rod_label_clip (Autodesk Fusion 360 design; units mm, degrees)
part number: 2026-09-05-07-00-16-324
Autodesk Fusion 360 part; units mm, degrees
sketch "Ring" plane through (0, 0, 0) normal (0, 1, 0) x (1, 0, 0)
  circle A0 centre (0, 0) radius 17.05
  circle A1 centre (0, 0) radius 19.45
  dimension "d32" = 34.1
  dimension "d33" = 38.9
  constraint coincident A0.centre A1.centre
  constraint concentric A0 A1
  measures "d32" diameter of A0
  measures "d33" diameter of A1
extrude "Ring (1)" add sketch "Ring" along normal mid plane 9
sketch "Mouth" plane through (0, 0, 0) normal (0, 1, 0) x (1, 0, 0)
  line L0 (0, 0) -> (42.3486, -24.45)
  line L1 (42.3486, -24.45) -> (-42.3486, -24.45)
  line L2 (-42.3486, -24.45) -> (0, 0)
  line L3 (0, 0) -> (0, -48.9) construction
  dimension "d36" = 48.9
  dimension "d37" = 60
  constraint coincident L0.start L2.end
  constraint vertical L3
  constraint symmetric L0 L2 L3
  measures "d36" distance of L0.start L0.end
  measures "d37" angle of L0 L3
extrude "Mouth (1)" cut sketch "Mouth" along normal mid plane 19
sketch "Stem" plane through (0, 0, 0) normal (0, 1, 0) x (1, 0, 0)
  line L0 (11.2039, 11.4854) -> (20.8457, 22.976)
  line L1 (20.8457, 22.976) -> (19.0072, 24.5187)
  line L2 (19.0072, 24.5187) -> (9.3653, 13.0281)
  line L3 (9.3653, 13.0281) -> (11.2039, 11.4854)
  dimension "d40" = 11.2039
  dimension "d41" = 11.4854
  dimension "d42" = 20.8457
  dimension "d43" = 22.976
  dimension "d44" = 19.0072
  dimension "d45" = 24.5187
  dimension "d46" = 9.3653
  dimension "d47" = 13.0281
  measures "d40" horizontal distance of origin L0.start
  measures "d41" vertical distance of origin L0.start
  measures "d42" horizontal distance of origin L0.end
  measures "d43" vertical distance of origin L0.end
  measures "d44" horizontal distance of origin L1.end
  measures "d45" vertical distance of origin L1.end
  measures "d46" horizontal distance of origin L2.end
  measures "d47" vertical distance of origin L2.end
extrude "Stem (1)" add sketch "Stem" along normal mid plane 9
sketch "Label face" plane through (0, 0, 0) normal (0, 1, 0) x (1, 0, 0)
  line L0 (20.8457, 22.976) -> (39.4865, 45.1913)
  line L1 (39.4865, 45.1913) -> (37.648, 46.734)
  line L2 (37.648, 46.734) -> (19.0072, 24.5187)
  line L3 (19.0072, 24.5187) -> (20.8457, 22.976)
  dimension "d50" = 20.8457
  dimension "d51" = 22.976
  dimension "d52" = 39.4865
  dimension "d53" = 45.1913
  dimension "d54" = 37.648
  dimension "d55" = 46.734
  dimension "d56" = 19.0072
  dimension "d57" = 24.5187
  measures "d50" horizontal distance of origin L0.start
  measures "d51" vertical distance of origin L0.start
  measures "d52" horizontal distance of origin L0.end
  measures "d53" vertical distance of origin L0.end
  measures "d54" horizontal distance of origin L1.end
  measures "d55" vertical distance of origin L1.end
  measures "d56" horizontal distance of origin L2.end
  measures "d57" vertical distance of origin L2.end
extrude "Label face (1)" add sketch "Label face" along normal mid plane 58
equation "clipWidth = 9.0 mm" comment "ring and stem width along the rod"
equation "faceWidth = 58.0 mm" comment "label face width along the rod"
equation "rodOuterDiameter = 33.4 mm" comment "rod the clip snaps onto"
equation "clipClearance = 0.7 mm" comment "diametral, so the clip slides"
equation "clipWall = 2.4 mm" comment "ring wall thickness"
equation "mouthHalfAngleDeg = 60.0 deg" comment "half the mouth opening"
equation "paddleThickness = 2.4 mm" comment "stem and label face thickness"
equation "stemEndRadius = 31.0 mm" comment "stem ends, label face begins"
equation "faceEndRadius = 60.0 mm" comment "outer edge of the label face"
equation "paddleAngleDeg = 50.0 deg" comment "paddle drop below horizontal"
equation "stemStartRadius = 16.0 mm" comment "stem starts inside the ring"
equation "d32 = rodOuterDiameter + clipClearance"
equation "d33 = rodOuterDiameter + clipClearance + 2 * clipWall"
equation "d34 = clipWidth"
equation "d36 = ( ( rodOuterDiameter + clipClearance + 2 * clipWall ) / 2 + 5 mm ) / cos(mouthHalfAngleDeg)"
equation "d37 = mouthHalfAngleDeg"
equation "d38 = clipWidth + 10 mm"
equation "d40 = stemStartRadius * cos(paddleAngleDeg) + paddleThickness / 2 * sin(paddleAngleDeg)"
equation "d41 = stemStartRadius * sin(paddleAngleDeg) - paddleThickness / 2 * cos(paddleAngleDeg)"
equation "d42 = stemEndRadius * cos(paddleAngleDeg) + paddleThickness / 2 * sin(paddleAngleDeg)"
equation "d43 = stemEndRadius * sin(paddleAngleDeg) - paddleThickness / 2 * cos(paddleAngleDeg)"
equation "d44 = stemEndRadius * cos(paddleAngleDeg) - paddleThickness / 2 * sin(paddleAngleDeg)"
equation "d45 = stemEndRadius * sin(paddleAngleDeg) + paddleThickness / 2 * cos(paddleAngleDeg)"
equation "d46 = stemStartRadius * cos(paddleAngleDeg) - paddleThickness / 2 * sin(paddleAngleDeg)"
equation "d47 = stemStartRadius * sin(paddleAngleDeg) + paddleThickness / 2 * cos(paddleAngleDeg)"
equation "d48 = clipWidth"
equation "d50 = stemEndRadius * cos(paddleAngleDeg) + paddleThickness / 2 * sin(paddleAngleDeg)"
equation "d51 = stemEndRadius * sin(paddleAngleDeg) - paddleThickness / 2 * cos(paddleAngleDeg)"
equation "d52 = faceEndRadius * cos(paddleAngleDeg) + paddleThickness / 2 * sin(paddleAngleDeg)"
equation "d53 = faceEndRadius * sin(paddleAngleDeg) - paddleThickness / 2 * cos(paddleAngleDeg)"
equation "d54 = faceEndRadius * cos(paddleAngleDeg) - paddleThickness / 2 * sin(paddleAngleDeg)"
equation "d55 = faceEndRadius * sin(paddleAngleDeg) + paddleThickness / 2 * cos(paddleAngleDeg)"
equation "d56 = stemEndRadius * cos(paddleAngleDeg) - paddleThickness / 2 * sin(paddleAngleDeg)"
equation "d57 = stemEndRadius * sin(paddleAngleDeg) + paddleThickness / 2 * cos(paddleAngleDeg)"
equation "d58 = faceWidth"
named bodies: "rod_label_clip"
